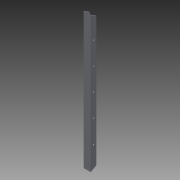
# Autodesk Inventor part: 24in C-Channel
Saved by Autodesk Inventor 2013 (Build 170138000, 138)
## iProperties
Created: 2013-01-12
Part Number: 24in C-Channel
Material: Generic
Document SubType Name: Modeling
Designer: carneeki
Density: 1 g/cm^3
Author: carneeki
Autodesk Inventor part; units mm, degrees
ref_plane "YZ Plane" through (0, 0, 0) normal (1, 0, 0) x (0, 1, 0)
ref_plane "XZ Plane" through (0, 0, 0) normal (0, 1, 0) x (-1, 0, 0)
ref_plane "XY Plane" through (0, 0, 0) normal (0, 0, 1) x (1, 0, 0)
sketch "Sketch1" plane through (0, 0, 0) normal (0, 0, 1) x (1, 0, 0)
  line L0 (-16, -12.5) -> (16, -12.5)
  line L1 (16, -12.5) -> (16, 12.5)
  line L2 (16, 12.5) -> (13, 12.5)
  line L3 (13, 12.5) -> (13, -9.5)
  line L4 (13, -9.5) -> (-13, -9.5)
  line L5 (-13, -9.5) -> (-13, 12.5)
  line L6 (-13, 12.5) -> (-16, 12.5)
  line L7 (-16, 12.5) -> (-16, -12.5)
  point P0 (0, 0)
  dimension "d0" = 32
  dimension "d1" = 25
  dimension "d2" = 3
  dimension "d3" = 90
  dimension "d4" = 22
  dimension "d5" = 26
  dimension "d6" = 22
  dimension "d7" = 3
  dimension "d8" = 25
  dimension "d10" = 12.5
  dimension "d11" = 16
  constraints: 16 end point, 5 parallel, 1 horizontal, 1 perpendicular
  measures "d0" distance of L0.start L0.end
  measures "d1" distance of L0.end L1.end
  measures "d2" distance of L1.end L2.end
  measures "d3" angle of L2 L1
  measures "d4" distance of L2.end L3.end
  measures "d5" distance of L3.end L4.end
  measures "d6" distance of L4.end L5.end
  measures "d7" distance of L5.end L6.end
  measures "d8" distance of L6.end L0.start
  measures "d10" distance from line of point (0, 0) L2
  measures "d11" distance from line of point (0, 0) L1
extrude "Extrusion1" add sketch "Sketch1" against normal blind 609.6
chamfer "Chamfer1" distance 25 angle 30 1 edges at (14.5, 12.5, 0) measured on face at (14.5, 12, 0)
chamfer "Chamfer2" distance 25 angle 30 1 edges at (14.5, 12.5, -609.6) measured on face at (14.5, 12, -609.6)
sketch "Sketch2" plane through (16, -12.5, 0) normal (1, 0, 0) x (0, 0, -1)
  line L0 (595.1662, 25) -> (609.6, 0) projected
  line L1 (14.4338, 25) -> (595.1662, 25) projected
  line L2 (602.3831, 12.5) -> (599.0481, 12.5)
  line L3 (508, 12.5) -> (101.6, 12.5) construction
  line L4 (101.6, 12.5) -> (203.2, 12.5) construction
  line L5 (203.2, 12.5) -> (304.8, 12.5) construction
  line L6 (304.8, 12.5) -> (406.4, 12.5) construction
  line L7 (406.4, 12.5) -> (508, 12.5) construction
  circle A0 centre (101.6, 12.5) radius 3.175
  circle A1 centre (203.2, 12.5) radius 3.175
  circle A2 centre (304.8, 12.5) radius 3.175
  circle A3 centre (406.4, 12.5) radius 3.175
  circle A4 centre (508, 12.5) radius 3.175
  line L8 (0, 12.5) -> (609.6, 12.5) construction
  point P0 (0, 0)
  dimension "d21" = 3.335
  dimension "d23" = 406.4
  dimension "d24" = 101.6
  dimension "d25" = 101.6
  dimension "d26" = 101.6
  dimension "d28" = 6.35
  dimension "d29" = 6.35
  dimension "d30" = 6.35
  dimension "d31" = 6.35
  dimension "d32" = 6.35
  dimension "d35" = 101.6
  dimension "d36" = 609.6
  dimension "d37" = 101.6
  dimension "d38" = 101.6
  constraints: 14 end point, 5 centre point, 5 coincident, 2 midpoint, 2 parallel, 2 point on line
  measures "d21" distance of L2.start L2.end
  measures "d23" distance of L3.start L3.end
  measures "d24" distance of L3.end L4.end
  measures "d25" distance of L4.end L5.end
  measures "d26" distance of L5.end L6.end
  measures "d28" diameter of A0
  measures "d29" diameter of A1
  measures "d30" diameter of A2
  measures "d31" diameter of A3
  measures "d32" diameter of A4
  measures "d35" distance of L3.end L8.start
  measures "d36" distance of point (0, 0) L0.end
  measures "d37" distance of L6.end L3.start
  measures "d38" distance of L8.end L3.start
extrude "Extrusion2" cut sketch "Sketch2" against normal blind 35
equation "\"d5\" = d0 - 2 * d2"
equation "\"d10\" = 0.5 * d1"
equation "\"d11\" = 0.5 * d0"
equation "\"d24\" = d35"
equation "\"d25\" = d24"
equation "\"d26\" = d24"
equation "\"d29\" = d28"
equation "\"d30\" = d28"
equation "\"d31\" = d28"
equation "\"d32\" = d28"
equation "\"d35\" = 0.166667 * d36"
equation "\"d37\" = d35"
body "Solid1"
